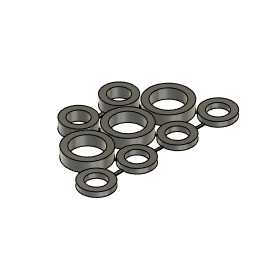
washers (Autodesk Fusion 360 design; units mm, degrees)
Autodesk Fusion 360 part; units mm, degrees
sketch "Sketch1" plane through (0, 0, 0) normal (0, 0, 1) x (1, 0, 0)
  circle A0 centre (35, 25) radius 4.25
  circle A1 centre (35, 25) radius 6
  circle A2 centre (35, 37.5) radius 6
  circle A3 centre (35, 37.5) radius 4.25
  circle A4 centre (35, 50) radius 6
  circle A5 centre (35, 50) radius 4.25
  circle A6 centre (26, 31.3) radius 4.5
  circle A7 centre (26, 31.3) radius 2.75
  circle A8 centre (26, 43.8) radius 4.5
  circle A9 centre (26, 43.8) radius 2.75
  circle A10 centre (44, 31.3) radius 4.5
  circle A11 centre (44, 31.3) radius 2.75
  circle A12 centre (44, 18.8) radius 2.75
  circle A13 centre (44, 18.8) radius 4.5
  circle A14 centre (44, 56.3) radius 4.5
  circle A15 centre (44, 56.3) radius 2.75
  circle A16 centre (44, 43.8) radius 4.5
  circle A17 centre (44, 43.8) radius 2.75
  line L0 (29.5225, 46.6003) -> (29.8899, 46.8556)
  line L1 (29.8449, 46.1381) -> (30.2075, 46.39)
  line L2 (34.7346, 44.0059) -> (34.7346, 43.4941)
  line L3 (35.433, 44.0156) -> (35.433, 43.2)
  line L4 (29.3463, 40.7913) -> (29.7769, 40.4528)
  line L5 (29.7769, 41.3535) -> (30.1629, 41.05)
  line L6 (29.7769, 34.5472) -> (29.373, 34.2787)
  line L7 (30.1629, 33.95) -> (29.8008, 33.7092)
  line L8 (34.6142, 31.5124) -> (34.6142, 30.9876)
  line L9 (35.2551, 31.5124) -> (35.2551, 30.9946)
  line L10 (29.4191, 28.3743) -> (29.8451, 28.0703)
  line L11 (29.7489, 28.8109) -> (30.1463, 28.5273)
  line L12 (39.7474, 28.6691) -> (40.1698, 28.9378)
  line L13 (40.0613, 28.2223) -> (40.4842, 28.4913)
  line L14 (39.9586, 34.1218) -> (40.3078, 33.8725)
  line L15 (40.3078, 34.7024) -> (40.7354, 34.3972)
  line L16 (40.3078, 22.2024) -> (40.7354, 21.8972)
  line L17 (39.9586, 21.6218) -> (40.3078, 21.3725)
  line L18 (43.6177, 26.8163) -> (43.6177, 23.2837)
  line L19 (44.3823, 26.8163) -> (44.3823, 23.2837)
  line L20 (43.6177, 39.3163) -> (43.6177, 35.7837)
  line L21 (44.1969, 39.3043) -> (44.1969, 35.7957)
  line L22 (40.0129, 41.7137) -> (39.59, 41.3642)
  line L23 (40.2163, 41.3642) -> (39.8367, 41.0505)
  line L24 (39.8151, 46.4203) -> (40.1765, 46.1729)
  line L25 (40.1765, 46.9662) -> (40.5614, 46.7028)
  line L26 (39.5856, 53.8694) -> (39.9958, 54.2466)
  line L27 (39.9958, 53.3229) -> (40.3584, 53.6564)
  line L28 (43.8974, 51.8012) -> (43.8974, 48.2988)
  line L29 (44.5001, 51.8279) -> (44.5001, 48.2721)
  line L30 (25.5335, 39.3242) -> (25.5335, 35.7758)
  line L31 (26.4665, 39.3242) -> (26.4665, 35.7758)
  dimension "d1" = 8.5
  dimension "d2" = 12
  dimension "d5" = 8.5
  dimension "d6" = 12
  dimension "d7" = 8.5
  dimension "d8" = 12
  dimension "d19" = 5.5
  dimension "d20" = 9
  dimension "d21" = 5.5
  dimension "d22" = 9
  dimension "d23" = 5.5
  dimension "d24" = 9
  dimension "d25" = 5.5
  dimension "d26" = 9
  dimension "d27" = 5.5
  dimension "d28" = 9
  dimension "d29" = 5.5
  dimension "d30" = 9
  constraint concentric A0 A1
  constraint concentric A2 A3
  constraint concentric A4 A5
  constraint concentric A6 A7
  constraint concentric A8 A9
  constraint concentric A12 A13
  constraint concentric A10 A11
  constraint concentric A16 A17
  constraint concentric A14 A15
  constraint coincident A8 L0.start
  constraint coincident A4 L0.end
  constraint coincident A8 L1.start
  constraint coincident A4 L1.end
  constraint parallel L0 L1
  constraint coincident A4 L2.start
  constraint coincident A2 L2.end
  constraint vertical L2
  constraint coincident A4 L3.start
  constraint parallel L2 L3
  constraint coincident A8 L4.start
  constraint coincident A2 L4.end
  constraint coincident A8 L5.start
  constraint coincident A2 L5.end
  constraint parallel L4 L5
  constraint coincident A2 L6.start
  constraint coincident A6 L6.end
  constraint coincident A2 L7.start
  constraint coincident A6 L7.end
  constraint parallel L6 L7
  constraint coincident A2 L8.start
  constraint coincident A1 L8.end
  constraint vertical L8
  constraint coincident A1 L9.end
  constraint parallel L8 L9
  constraint coincident A6 L10.start
  constraint coincident A1 L10.end
  constraint coincident A6 L11.start
  constraint coincident A1 L11.end
  constraint parallel L10 L11
  constraint coincident A1 L12.start
  constraint coincident A10 L12.end
  constraint coincident A1 L13.start
  constraint coincident A10 L13.end
  constraint parallel L12 L13
  constraint coincident A2 L14.start
  constraint coincident A10 L14.end
  constraint parallel L11 L14
  constraint coincident A2 L15.start
  constraint coincident A10 L15.end
  constraint parallel L14 L15
  constraint coincident A1 L16.start
  constraint coincident A13 L16.end
  constraint parallel L15 L16
  constraint coincident A1 L17.start
  constraint coincident A13 L17.end
  constraint parallel L16 L17
  constraint coincident A10 L18.start
  constraint coincident A13 L18.end
  constraint vertical L18
  constraint coincident A10 L19.start
  constraint coincident A13 L19.end
  constraint parallel L18 L19
  constraint coincident A16 L20.start
  constraint coincident A10 L20.end
  constraint parallel L19 L20
  constraint coincident A16 L21.start
  constraint coincident A10 L21.end
  constraint vertical L21
  constraint coincident A16 L22.start
  constraint coincident A2 L22.end
  constraint coincident A16 L23.start
  constraint coincident A2 L23.end
  constraint parallel L22 L23
  constraint coincident A4 L24.start
  constraint coincident A16 L24.end
  constraint coincident A4 L25.start
  constraint coincident A16 L25.end
  constraint parallel L24 L25
  constraint coincident A4 L26.start
  constraint coincident A14 L26.end
  constraint coincident A4 L27.start
  constraint coincident A14 L27.end
  constraint parallel L26 L27
  constraint coincident A14 L28.start
  constraint coincident A16 L28.end
  constraint vertical L28
  constraint coincident A14 L29.start
  constraint coincident A16 L29.end
  constraint parallel L28 L29
  constraint coincident A8 L30.start
  constraint coincident A6 L30.end
  constraint parallel L29 L30
  constraint coincident A8 L31.start
  constraint coincident A6 L31.end
  constraint parallel L30 L31
  measures "d1" diameter of A0
  measures "d2" diameter of A1
  measures "d5" diameter of A3
  measures "d6" diameter of A2
  measures "d7" diameter of A5
  measures "d8" diameter of A4
  measures "d19" diameter of A7
  measures "d20" diameter of A6
  measures "d21" diameter of A9
  measures "d22" diameter of A8
  measures "d23" diameter of A12
  measures "d24" diameter of A13
  measures "d25" diameter of A11
  measures "d26" diameter of A10
  measures "d27" diameter of A17
  measures "d28" diameter of A16
  measures "d29" diameter of A15
  measures "d30" diameter of A14
extrude "Extrude1" add sketch "Sketch1" along normal blind 3 contours A1 | A2 | A6 | A8 | A4 makes body 1 at (40.9702, 36.9026, 1) makes body 2 at (30.4776, 30.8519, 1) makes body 3 at (40.9702, 50.5974, 2) makes body 4 at (30.4776, 44.2481, 2) makes body 5 at (40.9702, 24.4026, 1)
extrude "Extrude2" add sketch "Sketch1" along normal blind 1.5 separate body contours A10 | A13 | A16 | A14 makes body 6 at (48.4776, 31.7481, 1) makes body 7 at (48.4776, 43.3519, 0.5) makes body 8 at (48.4776, 18.3519, 0.5) makes body 9 at (48.4776, 56.7481, 1)
extrude "Extrude3" add sketch "Sketch1" along normal blind 0.2 contours A1 A10 L12 L13 | A1 A13 L16 L17 | A1 A2 L8 L9 | A10 A13 L18 L19 | A1 A6 L10 L11 | A2 A10 L14 L15 | A6 A8 L30 L31 | A2 A6 L6 L7 | A10 A16 L20 L21 | A4 A8 L0 L1 | A2 A8 L4 L5 | A2 A16 L22 L23 | A14 A16 L28 L29 | A4 A14 L26 L27 | A2 A4 L2 L3 | A4 A16 L24 L25 bodies 1 2 3 4 5 6 7 8 9
